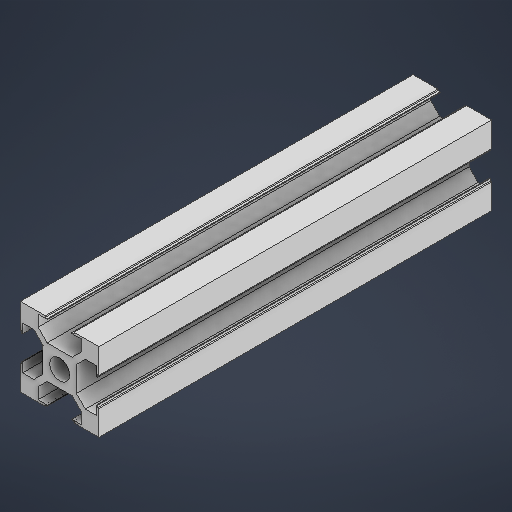
# Autodesk Inventor part: 铝方管2020x60
Saved by Autodesk Inventor 2025 (Build 290162000, 162)
## iProperties
Created: 2025-06-18
Part Number: 铝方管2020x60
Material: 常规
Document SubType Name: Modeling
Designer: XH
Density: 1 g/cm^3
Appearance: 默认
Author: XH
Autodesk Inventor part; units mm, degrees
ref_plane "YZ Plane" through (0, 0, 0) normal (1, 0, 0) x (0, 1, 0)
ref_plane "XZ Plane" through (0, 0, 0) normal (0, 1, 0) x (-1, 0, 0)
ref_plane "XY Plane" through (0, 0, 0) normal (0, 0, 1) x (1, 0, 0)
sketch "草图1" plane through (0, 0, 0) normal (0, 0, 1) x (1, 0, 0)
  line L0 (10, -10) -> (-10, -10)
  line L1 (-10, -10) -> (-10, 10)
  line L2 (-10, 10) -> (10, 10)
  line L3 (10, 10) -> (10, -10)
  line L4 (10, -10) -> (-10, 10) construction
  line L5 (-10, -10) -> (10, 10) construction
  point P0 (0, 0)
  dimension "d0" = 20
  dimension "d1" = 20
  constraints: 12 end point, 2 midpoint, 2 parallel, 1 horizontal, 1 perpendicular
  measures "d0" distance of L1.end L2.end
  measures "d1" distance of L0.end L1.end
extrude "拉伸1" add sketch "草图1" along normal blind 100
sketch "草图2" plane through (0, 0, 100) normal (0, 0, 1) x (1, 0, 0)
  line L0 (-10.3453, 3.6494) -> (-10.3453, 10.3451)
  line L1 (-10.3453, 3.0994) -> (-10.3453, 10.3451)
  line L2 (-10.3453, 10.3451) -> (-10.3453, -10.0013)
  line L3 (-10.3453, 5.4994) -> (-10.3453, 10.3451)
  line L4 (-3.6495, 9.6435) -> (-3.0995, 9.6435)
  line L5 (-5.4995, 12.01) -> (-5.4995, 5.4994)
  line L6 (-3.0995, 10.3451) -> (-3.0995, 9.4451)
  line L7 (-5.4995, 9.4451) -> (0.0005, 9.4451)
  line L8 (-3.6495, 10.3451) -> (-3.6495, 9.4451)
  circle A0 centre (0.0005, -0.0006) radius 2.55
  line L9 (-5.4995, 10.3451) -> (-5.4995, 5.4994)
  line L10 (-10.3453, 10.3451) -> (-5.4995, 10.3451)
  line L11 (-5.4995, 5.4994) -> (-10.3453, 5.4994)
  line L12 (-4.2453, 4.2451) -> (-4.2453, -0.0006)
  line L13 (-10.3453, 10.3451) -> (-3.6495, 10.3451)
  line L14 (-10.3453, 10.3451) -> (-3.0995, 10.3451)
  line L15 (-11.061, -0.0006) -> (0.0005, -0.0006)
  line L16 (-1.0602, -0.0006) -> (-10.3453, 9.2845)
  line L17 (-10.3453, 10.3451) -> (0.0005, -0.0006)
  line L18 (0.0005, 1.06) -> (-9.2846, 10.3451)
  line L19 (0.0005, -0.0006) -> (0.0005, 11.5494)
  line L20 (10.0005, 10.3451) -> (-10.3453, 10.3451)
  line L21 (0.0005, 4.2451) -> (-4.2453, 4.2451)
  point P0 (0, 0)
  point P1 (-3.0995, 9.8951)
  point P2 (-5.4995, 6.56)
  point P3 (-3.1846, 4.2451)
  point P4 (0.0005, 10.3451)
  point P5 (-3.0995, 10.3451)
  dimension "d4" = 5.1
  dimension "d5" = 6.1
  dimension "d6" = 1.5
  dimension "d7" = 5.5
  dimension "d8" = 0.9
  dimension "d9" = 3.1
  dimension "d10" = 3.65
  constraints: 44 end point, 12 point on line, 7 perpendicular, 5 horizontal, 5 parallel, 2 coincident, 2 symmetric about line, 1 centre point, 1 midpoint, 1 vertical
  measures "d4" diameter of A0
  measures "d5" distance between parallel lines of L12 L2
  measures "d6" distance between parallel lines of L16 L18
  measures "d7" distance between parallel lines of L5 L19
  measures "d8" distance between parallel lines of L20 L7
  measures "d9" distance from line of point (-3.1, 9.895) L19
  measures "d10" distance between parallel lines of L8 L19
extrude "拉伸2" cut sketch "草图2" against normal blind 205.75 contours L5 L7 L19 L21 L18 | L16 L15 A0 | A0 L17 L15 L16 | L15 L19 A0 | A0 L18 L19 L17 | L14 L6 L4 L8 | A0 L19 L18 | L20 L19 L7 L6
mirror "镜像1" about plane through (0.0005, 10.3451, 100) normal (-1, 0, 0) of "拉伸2"
pattern_circular "环形阵列1" count 4 over 360 about axis through (0.0005, -0.0006, 100) along (0, 0, -1) of "拉伸2", "镜像1"
